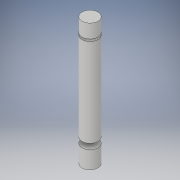
# Autodesk Inventor part: RollerFull
Saved by Autodesk Inventor 2017 (Build 210142000, 142)
## iProperties
Created: 2017-05-06
Part Number: RollerFull
Material: Generic
Document SubType Name: Modeling
Designer: User
Density: 1 g/cm^3
Appearance: Default
Author: User
Autodesk Inventor part; units mm, degrees
ref_plane "YZ Plane" through (0, 0, 0) normal (1, 0, 0) x (0, 1, 0)
ref_plane "XZ Plane" through (0, 0, 0) normal (0, 1, 0) x (-1, 0, 0)
ref_plane "XY Plane" through (0, 0, 0) normal (0, 0, 1) x (1, 0, 0)
sketch "Sketch2" plane through (0, 0, 0) normal (1, 0, 0) x (0, 1, 0)
  line L0 (0, 0) -> (457.2, 0)
  line L1 (457.2, 0) -> (457.2, -57.15)
  line L2 (457.2, -57.15) -> (0, -57.15)
  line L3 (0, -57.15) -> (0, 0)
  line L4 (407.543, 0) -> (400.05, 0)
  line L5 (400.05, 0) -> (400.05, -57.15)
  line L6 (400.05, -57.15) -> (407.543, -57.15)
  line L7 (407.543, -57.15) -> (407.543, 0)
  line L8 (82.55, 0) -> (62.865, 0)
  line L9 (62.865, 0) -> (62.865, -57.15)
  line L10 (62.865, -57.15) -> (82.55, -57.15)
  line L11 (82.55, -57.15) -> (82.55, 0)
  dimension "d3" = 457.2
  dimension "d4" = 57.15
  dimension "d5" = 7.493
  dimension "d6" = 49.657
  dimension "d7" = 19.685
  dimension "d8" = 62.865
  constraints: 24 end point, 6 parallel, 4 point on line, 3 horizontal, 3 perpendicular
  measures "d3" distance of L1.end L2.end
  measures "d4" distance of L0.end L1.end
  measures "d5" distance of L6.end L5.end
  measures "d6" distance between parallel lines of L1 L7
  measures "d7" distance of L10.end L9.end
  measures "d8" distance between parallel lines of L3 L9
extrude "Extrusion2" add sketch "Sketch2" along normal blind 57.15 contours L0 L9 L2 L3 | L0 L5 L2 L11 | L0 L1 L2 L7
sketch "Sketch3" plane through (0, 457.2, 0) normal (0, 1, 0) x (1, 0, 0)
  circle A0 centre (28.575, 28.575) radius 28.575
  line L0 (0, 57.15) -> (0, 0) projected
  line L1 (0, 0) -> (57.15, 0) projected
  line L2 (57.15, 57.15) -> (57.15, 0) projected
  line L3 (0, 57.15) -> (57.15, 57.15) projected
  dimension "d11" = 57.15
  dimension "d12" = 28.575
  dimension "d13" = 28.575
  constraints: 1 centre point
  measures "d11" diameter of A0
  measures "d12" distance from line of A0.centre L0
  measures "d13" distance from line of L1 A0.centre
extrude "Extrusion3" cut sketch "Sketch3" against normal blind 457.2 contours L2 L1 A0 | A0 L3 L2 | A0 L0 L3 | L1 L0 A0
body "Solid2"
